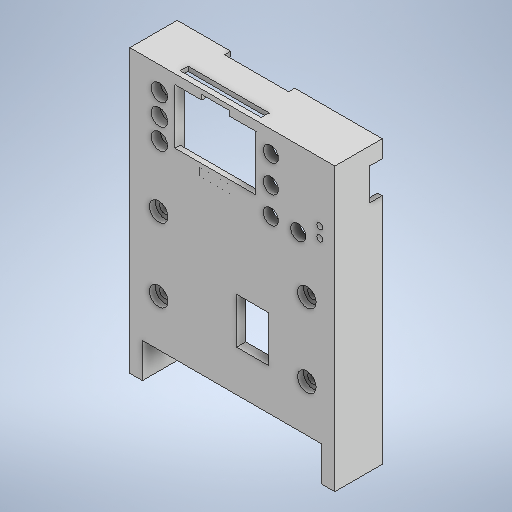
# Autodesk Inventor part: TES_Controller_V1_Case_Top
Saved by Autodesk Inventor 2025 (Build 290162000, 162)
## iProperties
Created: 2025-08-31
Part Number: TES_Controller_V1_Case_Top
Material: 常规
Document SubType Name: Modeling
Designer: 95052
Density: 1 g/cm^3
Appearance: 默认
Author: 95052
Autodesk Inventor part; units mm, degrees
ref_plane "YZ Plane" through (0, 0, 0) normal (1, 0, 0) x (0, 1, 0)
ref_plane "XZ Plane" through (0, 0, 0) normal (0, 1, 0) x (-1, 0, 0)
ref_plane "XY Plane" through (0, 0, 0) normal (0, 0, 1) x (1, 0, 0)
sketch "草图22" plane through (0, 0, 0) normal (0, 0, 1) x (1, 0, 0)
  line L0 (32.055, -44.6465) -> (-32.055, -44.6465)
  line L1 (-32.055, -44.6465) -> (-32.055, 44.6465)
  line L2 (-32.055, 44.6465) -> (32.055, 44.6465)
  line L3 (32.055, 44.6465) -> (32.055, -44.6465)
  line L4 (32.055, -44.6465) -> (-32.055, 44.6465) construction
  line L5 (-32.055, -44.6465) -> (32.055, 44.6465) construction
  line L6 (24.394, -19.5595) -> (-24.107, -19.5595) construction
  line L7 (-24.107, -19.5595) -> (-24.107, 4.4405) construction
  line L8 (-24.107, 4.4405) -> (24.394, 4.4405) construction
  line L9 (24.394, 4.4405) -> (24.394, -19.5595) construction
  line L10 (24.394, -19.5595) -> (-24.107, 4.4405) construction
  line L11 (-24.107, -19.5595) -> (24.394, 4.4405) construction
  circle A0 centre (-24.107, 4.4405) radius 1.7
  circle A1 centre (-24.107, -19.5595) radius 1.7
  circle A2 centre (24.394, -19.5595) radius 1.7
  circle A3 centre (24.394, 4.4405) radius 1.7
  point P0 (0, 0)
  point P1 (-14.525, 44.6465)
  point P2 (3.476, 44.6465)
  point P3 (0.1435, -7.5595)
  dimension "d101" = 89.293
  dimension "d102" = 64.11
  dimension "d103" = 7.661
  dimension "d104" = 7.948
  dimension "d105" = 25.087
  dimension "d106" = 40.206
  dimension "d107" = 17.53
  dimension "d108" = 28.579
  dimension "d109" = 3.4
  dimension "d110" = 3.4
  dimension "d111" = 3.4
  dimension "d112" = 3.4
  constraints: 24 end point, 4 centre point, 4 coincident, 4 midpoint, 4 parallel, 2 horizontal, 2 perpendicular, 2 point on line
  measures "d101" distance of L2.end L0.start
  measures "d102" distance of L0.start L0.end
  measures "d103" distance between parallel lines of L3 L9
  measures "d104" distance between parallel lines of L1 L7
  measures "d105" distance between parallel lines of L0 L6
  measures "d106" distance between parallel lines of L2 L8
  measures "d107" distance from line of L1 point (-14.525, 44.646)
  measures "d108" distance from line of L3 point (3.476, 44.646)
  measures "d109" diameter of A0
  measures "d110" diameter of A1
  measures "d111" diameter of A2
  measures "d112" diameter of A3
extrude "拉伸18" add sketch "草图22" along normal blind 1
sketch "草图23" plane through (0, 0, 1) normal (0, 0, 1) x (1, 0, 0)
  circle A0 centre (-24.107, 4.4405) radius 1.7 projected
  circle A1 centre (24.394, 4.4405) radius 1.7 projected
  circle A2 centre (24.394, -19.5595) radius 1.7 projected
  circle A3 centre (-24.107, -19.5595) radius 1.7 projected
  line L0 (32.055, 44.6465) -> (-32.055, 44.6465) projected
  line L1 (-32.055, -44.6465) -> (32.055, -44.6465) projected
  line L2 (-32.055, 44.6465) -> (32.055, 44.6465)
  line L3 (32.055, 44.6465) -> (32.055, -44.6465)
  line L4 (32.055, -44.6465) -> (-32.055, -44.6465)
  line L5 (-32.055, -44.6465) -> (-32.055, 44.6465)
  circle A4 centre (24.394, 4.4405) radius 3.05
  circle A5 centre (24.394, -19.5595) radius 1.7 projected
  circle A6 centre (24.394, -19.5595) radius 3.05
  circle A7 centre (-24.107, -19.5595) radius 3.05
  circle A8 centre (-24.107, 4.4405) radius 3.05
  point P0 (0, 0)
  dimension "d164" = 6.1
  constraints: 8 coincident, 8 end point, 4 centre point, 3 equal radius, 2 parallel, 1 horizontal, 1 perpendicular
  measures "d164" diameter of A4
extrude "拉伸19" add sketch "草图23" along normal blind 2 contours L3 L1 L5 L0
sketch "草图25" plane through (0, 0, 3) normal (0, 0, 1) x (1, 0, 0)
  circle A0 centre (-23.869, 38.3445) radius 2.7
  circle A1 centre (-23.869, 31.3595) radius 2.7
  circle A2 centre (-23.869, 24.5015) radius 2.7
  line L0 (32.055, 44.6465) -> (-32.055, 44.6465) projected
  line L1 (-32.055, 44.6465) -> (-32.055, -44.6465) projected
  circle A3 centre (12.608, 39.1095) radius 2.5
  line L2 (32.055, -44.6465) -> (32.055, 44.6465) projected
  circle A4 centre (12.608, 30.2185) radius 2.5
  circle A5 centre (12.608, 21.3885) radius 2.5
  circle A6 centre (21.582, 21.3885) radius 2.5
  circle A7 centre (28.639, 26.6255) radius 1
  circle A8 centre (28.639, 23.2155) radius 1
  line L3 (7.225, 20.5575) -> (-18.275, 20.5575) construction
  line L4 (-18.275, 20.5575) -> (-18.275, 47.0575) construction
  line L5 (-18.275, 47.0575) -> (7.225, 47.0575) construction
  line L6 (7.225, 47.0575) -> (7.225, 20.5575) construction
  line L7 (-18.775, 25.0575) -> (7.725, 25.0575)
  line L8 (7.725, 25.0575) -> (7.725, 43.0575)
  line L9 (-18.775, 43.0575) -> (-18.775, 25.0575)
  line L10 (-10.025, 43.0575) -> (-10.025, 47.0575)
  line L11 (-10.025, 47.0575) -> (-5.525, 47.0575)
  line L12 (-1.025, 43.0575) -> (-1.025, 47.0575)
  line L13 (-1.025, 47.0575) -> (-5.525, 47.0575)
  line L14 (7.725, 43.0575) -> (-1.025, 43.0575)
  line L15 (-10.025, 43.0575) -> (-18.775, 43.0575)
  point P0 (0, 0)
  point P1 (-5.525, 21.0575)
  point P2 (-5.525, 20.5575)
  dimension "d123" = 5.4
  dimension "d124" = 5.4
  dimension "d125" = 5.4
  dimension "d126" = 6.302
  dimension "d127" = 8.186
  dimension "d128" = 8.186
  dimension "d129" = 8.186
  dimension "d130" = 13.287
  dimension "d131" = 20.145
  dimension "d132" = 5.537
  dimension "d133" = 19.447
  dimension "d134" = 5
  dimension "d135" = 5
  dimension "d136" = 14.428
  dimension "d137" = 19.447
  dimension "d138" = 5
  dimension "d139" = 19.447
  dimension "d140" = 23.258
  dimension "d141" = 5
  dimension "d142" = 23.258
  dimension "d143" = 10.473
  dimension "d144" = 2
  dimension "d145" = 2
  dimension "d146" = 3.416
  dimension "d147" = 3.416
  dimension "d148" = 18.021
  dimension "d149" = 3.41
  dimension "d150" = 26.53
  dimension "d151" = 23.589
  dimension "d152" = 0.5
  dimension "d153" = 26.53
  dimension "d154" = 26.5
  dimension "d155" = 25.5
  dimension "d156" = 4.5
  dimension "d158" = 0.5
  dimension "d159" = 0.5
  constraints: 26 end point, 9 centre point, 5 parallel, 2 collinear, 2 horizontal, 2 perpendicular, 1 midpoint
  measures "d123" diameter of A0
  measures "d124" diameter of A1
  measures "d125" diameter of A2
  measures "d126" distance from line of L0 A0.centre
  measures "d127" distance from line of L1 A0.centre
  measures "d128" distance from line of L1 A1.centre
  measures "d129" distance from line of L1 A2.centre
  measures "d130" distance from line of L0 A1.centre
  measures "d131" distance from line of L0 A2.centre
  measures "d132" distance from line of L0 A3.centre
  measures "d133" distance from line of L2 A3.centre
  measures "d134" diameter of A3
  measures "d135" diameter of A4
  measures "d136" distance from line of L0 A4.centre
  measures "d137" distance from line of L2 A4.centre
  measures "d138" diameter of A5
  measures "d139" distance from line of L2 A5.centre
  measures "d140" distance from line of L0 A5.centre
  measures "d141" diameter of A6
  measures "d142" distance from line of L0 A6.centre
  measures "d143" distance from line of L2 A6.centre
  measures "d144" diameter of A7
  measures "d145" diameter of A8
  measures "d146" distance from line of L2 A7.centre
  measures "d147" distance from line of L2 A8.centre
  measures "d148" distance from line of L0 A7.centre
  measures "d149" distance of A7.centre A8.centre
  measures "d150" distance from line of L1 point (-5.525, 21.058)
  measures "d151" distance from line of L0 point (-5.525, 21.058)
  measures "d152" distance from line of point (-5.525, 21.058) L3
  measures "d153" distance from line of L1 point (-5.525, 20.558)
  measures "d154" distance of L3.end L4.end
  measures "d155" distance of L3.start L3.end
  measures "d156" distance between parallel lines of L3 L7
  measures "d158" distance between parallel lines of L4 L9
  measures "d159" distance between parallel lines of L6 L8
extrude "拉伸21" cut sketch "草图25" against normal up to next
sketch "草图26" plane through (0, 0, 3) normal (0, 0, 1) x (1, 0, 0)
  circle A0 centre (-24.107, 4.4405) radius 1.7 projected
  circle A1 centre (-24.107, -19.5595) radius 1.7 projected
  circle A2 centre (24.394, 4.4405) radius 1.7 projected
  circle A3 centre (24.394, -19.5595) radius 1.7 projected
  line L0 (1.394, -6.2595) -> (11.894, -6.2595)
  line L1 (11.894, -6.2595) -> (11.894, -21.2595)
  line L2 (11.894, -21.2595) -> (1.394, -21.2595)
  line L3 (1.394, -21.2595) -> (1.394, -6.2595)
  line L4 (-24.107, -19.5595) -> (24.394, -19.5595) construction
  line L5 (32.055, -44.6465) -> (32.055, 44.6465) construction
  line L6 (24.394, -21.2595) -> (-24.107, -21.2595) construction
  point P0 (0, 0)
  dimension "d165" = 12.5
  dimension "d166" = 23
  dimension "d167" = 15
  constraints: 12 end point, 2 horizontal, 2 parallel, 2 perpendicular, 2 vertical alignment, 1 collinear, 2 other
  measures "d165" distance from line of L1 L4.end
  measures "d166" distance from line of L4.end L3
  measures "d167" distance between parallel lines of L2 L0
extrude "拉伸22" cut sketch "草图26" against normal through all contours L0 L1 L2 L3
sketch "草图27" plane through (0, 0, 0) normal (0, 0, -1) x (-1, 0, 0)
  line L0 (10.855, 21.0575) -> (0.195, 21.0575)
  line L1 (0.195, 21.0575) -> (0.195, 23.5575)
  line L2 (0.195, 23.5575) -> (10.855, 23.5575)
  line L3 (10.855, 23.5575) -> (10.855, 21.0575)
  line L4 (10.025, 44.6465) -> (32.055, 44.6465) projected
  line L5 (32.055, 44.6465) -> (32.055, -44.6465) projected
  point P0 (0, 0)
  dimension "d170" = 23.589
  dimension "d171" = 21.089
  dimension "d172" = 21.2
  dimension "d173" = 31.86
  constraints: 8 end point, 2 parallel, 1 horizontal, 1 perpendicular
  measures "d170" distance between parallel lines of L4 L0
  measures "d171" distance between parallel lines of L4 L2
  measures "d172" distance between parallel lines of L5 L3
  measures "d173" distance between parallel lines of L5 L1
extrude "拉伸23" cut sketch "草图27" against normal blind 2.8
sketch "草图28" plane through (0, 0, 3) normal (0, 0, 1) x (1, 0, 0)
  line L0 (-32.055, -44.6465) -> (32.055, -44.6465) projected
  line L1 (-29.408, -44.6465) -> (29.212, -44.6465)
  line L2 (29.212, -44.6465) -> (29.212, -34.7635)
  line L3 (29.212, -34.7635) -> (-29.408, -34.7635)
  line L4 (-29.408, -34.7635) -> (-29.408, -44.6465)
  line L5 (32.055, -44.6465) -> (32.055, 44.6465) projected
  line L6 (-32.055, 44.6465) -> (-32.055, -44.6465) projected
  point P0 (0, 0)
  point P1 (29.212, -44.6465)
  dimension "d176" = 2.843
  dimension "d177" = 2.647
  dimension "d178" = 9.883
  constraints: 8 end point, 2 parallel, 1 horizontal, 1 perpendicular, 1 point on line
  measures "d176" distance between parallel lines of L2 L5
  measures "d177" distance between parallel lines of L6 L4
  measures "d178" distance between parallel lines of L0 L3
extrude "拉伸24" cut sketch "草图28" against normal through all
sketch "草图29" plane through (0, 0, 0) normal (0, 0, -1) x (-1, 0, 0)
  line L0 (29.408, -34.7635) -> (-29.212, -34.7635) projected
  line L1 (29.408, -34.7635) -> (-29.212, -34.7635)
  line L2 (-29.212, -34.7635) -> (-29.212, -32.7635)
  line L3 (-29.212, -32.7635) -> (29.408, -32.7635)
  line L4 (29.408, -32.7635) -> (29.408, -34.7635)
  point P0 (0, 0)
  point P1 (-29.212, -34.7635)
  dimension "d181" = 2
  constraints: 8 end point, 2 parallel, 1 horizontal, 1 perpendicular
  measures "d181" distance of L1.end L2.end
extrude "拉伸25" add sketch "草图29" along normal blind 3
sketch "草图30" plane through (0, 0, 0) normal (0, 0, -1) x (-1, 0, 0)
  line L0 (29.408, -32.7635) -> (29.408, -34.7635) projected
  line L1 (32.055, 44.6465) -> (32.055, -44.6465) projected
  line L2 (29.408, -32.7635) -> (32.055, -32.7635)
  line L3 (32.055, -32.7635) -> (32.055, -44.6465)
  line L4 (32.055, -44.6465) -> (29.408, -44.6465)
  line L5 (29.408, -44.6465) -> (29.408, -32.7635)
  line L6 (-29.212, -34.7635) -> (-29.212, -32.7635) projected
  line L7 (-32.055, -44.6465) -> (-32.055, 44.6465) projected
  line L8 (-29.212, -32.7635) -> (-32.055, -32.7635)
  line L9 (-32.055, -32.7635) -> (-32.055, -44.6465)
  line L10 (-32.055, -44.6465) -> (-29.212, -44.6465)
  line L11 (-29.212, -44.6465) -> (-29.212, -32.7635)
  point P0 (0, 0)
  constraints: 16 end point, 4 parallel, 2 horizontal, 2 perpendicular
extrude "拉伸26" add sketch "草图30" along normal blind 11.5
sketch "草图31" plane through (0, 0, 0) normal (0, 0, -1) x (-1, 0, 0)
  line L0 (-32.055, -32.7635) -> (-32.055, 44.6465) projected
  line L1 (32.055, 44.6465) -> (32.055, -32.7635) projected
  line L2 (-33.555, 44.6465) -> (-33.555, -44.6465)
  line L3 (-32.055, -44.6465) -> (-32.055, 44.6465)
  line L4 (33.555, 44.6465) -> (33.555, -44.6465)
  line L5 (32.055, -44.6465) -> (32.055, 44.6465)
  line L6 (-32.055, 44.6465) -> (32.055, 44.6465)
  line L7 (33.555, 44.6465) -> (33.555, 46.1465)
  line L8 (33.555, 46.1465) -> (-33.555, 46.1465)
  line L9 (-33.555, 46.1465) -> (-33.555, 44.6465)
  line L10 (29.408, -44.6465) -> (32.055, -44.6465)
  line L11 (33.555, -44.6465) -> (33.555, -46.1465)
  line L12 (33.555, -46.1465) -> (29.408, -46.1465)
  line L13 (29.408, -46.1465) -> (29.408, -44.6465)
  line L14 (-32.055, -44.6465) -> (-29.212, -44.6465)
  line L15 (-29.212, -44.6465) -> (-29.212, -46.1465)
  line L16 (-29.212, -46.1465) -> (-33.555, -46.1465)
  line L17 (-33.555, -46.1465) -> (-33.555, -44.6465)
  point P0 (0, 0)
  point P1 (-32.055, 44.6465)
  point P2 (32.055, -32.7635)
  dimension "d188" = 1.5
  dimension "d202" = 1.5
  constraints: 32 end point, 8 parallel, 3 horizontal, 3 perpendicular, 3 point on line
  measures "d188" distance of L7.end L7.start
  measures "d202" distance of L14.end L15.end
extrude "拉伸27" add sketch "草图31" along normal blind 11.5 and the other way blind 3
sketch "草图32" plane through (-33.555, 46.1465, -11.5) normal (0, 1, 0) x (1, 0, 0)
  line L0 (14.78, -11.5) -> (41.28, -11.5) projected
  line L1 (41.28, -11.5) -> (14.78, -11.5)
  line L2 (14.78, -11.5) -> (14.78, -10.2)
  line L3 (14.78, -10.2) -> (41.28, -10.2)
  line L4 (41.28, -10.2) -> (41.28, -11.5)
  point P0 (33.555, -11.5)
  dimension "d193" = 1.3
  constraints: 8 end point, 2 parallel, 1 horizontal, 1 perpendicular
  measures "d193" distance of L1.end L2.end
extrude "拉伸28" cut sketch "草图32" against normal blind 11
sketch "草图33" plane through (-33.555, 46.1465, -11.5) normal (0, 1, 0) x (1, 0, 0)
  line L0 (65.61, 0) -> (1.5, 0) projected
  line L1 (17.53, 0) -> (38.5, 0)
  line L2 (38.5, 0) -> (38.5, -1)
  line L3 (38.5, -1) -> (17.53, -1)
  line L4 (17.53, -1) -> (17.53, 0)
  point P0 (33.555, -11.5)
  dimension "d196" = 16.03
  dimension "d197" = 37
  dimension "d198" = 1
  constraints: 8 end point, 2 parallel, 1 horizontal, 1 perpendicular, 1 point on line
  measures "d196" distance from line of L4 L0.end
  measures "d197" distance from line of L0.end L2
  measures "d198" distance between parallel lines of L0 L3
extrude "拉伸29" cut sketch "草图33" against normal blind 11
sketch "草图34" plane through (0, 0, 0) normal (0, 0, -1) x (-1, 0, 0)
  line L0 (18.775, 44.6465) -> (32.055, 44.6465) projected
  line L1 (18.775, 21.0575) -> (18.775, 44.6465)
  line L2 (-7.725, 44.6465) -> (-7.725, 21.0575)
  line L3 (10.855, 21.0575) -> (0.195, 21.0575) projected
  line L4 (18.775, 20.5575) -> (-7.725, 20.5575)
  line L5 (-7.725, 46.1465) -> (18.775, 46.1465)
  line L6 (-7.725, 44.6465) -> (-7.725, 46.1465)
  line L7 (-7.725, 46.1465) -> (-7.725, 44.6465) projected
  line L8 (-7.725, 21.0575) -> (-7.725, 20.5575)
  line L9 (18.775, 21.0575) -> (18.775, 20.5575)
  line L10 (18.775, 44.6465) -> (18.775, 46.1465)
  line L11 (-4.945, 46.1465) -> (16.025, 46.1465) projected
  point P0 (0, 0)
  constraints: 16 end point, 3 point on line, 2 parallel, 1 collinear, 1 perpendicular
extrude "拉伸30" cut sketch "草图34" against normal blind 1.3
sketch "草图35" plane through (33.555, -46.1465, -11.5) normal (1, 0, 0) x (0, 0, -1)
  line L0 (0, 90.793) -> (0, 13.383) projected
  line L1 (0, 86.614) -> (-3, 86.614)
  line L2 (-3, 86.614) -> (-3, 76.174)
  line L3 (-3, 76.174) -> (0, 76.174)
  line L4 (0, 76.174) -> (0, 86.614)
  line L5 (-11.5, 90.793) -> (0, 90.793) projected
  point P0 (-11.5, 46.1465)
  point P1 (-1.5, 86.614)
  point P2 (0, 76.174)
  point P3 (-0.0335, 85.614)
  dimension "d206" = 4.179
  dimension "d207" = 14.619
  dimension "d208" = 3
  constraints: 8 end point, 2 parallel, 1 horizontal, 1 midpoint, 1 perpendicular, 1 point on line
  measures "d206" distance from line of L5 point (-1.5, 86.614)
  measures "d207" distance between parallel lines of L5 L3
  measures "d208" distance between parallel lines of L0 L2
extrude "拉伸31" cut sketch "草图35" against normal up to surface (1.5 mm away)
sketch "草图37" plane through (0, 0, 0) normal (0, 0, -1) x (-1, 0, 0)
  circle A0 centre (24.107, 4.4405) radius 1.7 projected
  circle A1 centre (24.107, 4.4405) radius 3
  circle A2 centre (24.107, -19.5595) radius 1.7 projected
  circle A3 centre (24.107, -19.5595) radius 3
  circle A4 centre (-24.394, 4.4405) radius 1.7 projected
  circle A5 centre (-24.394, 4.4405) radius 3
  circle A6 centre (-24.394, -19.5595) radius 1.7 projected
  circle A7 centre (-24.394, -19.5595) radius 3
  point P0 (0, 0)
  dimension "d213" = 6
  dimension "d214" = 6
  dimension "d215" = 6
  dimension "d216" = 6
  constraints: 4 centre point, 4 coincident
  measures "d213" diameter of A1
  measures "d214" diameter of A3
  measures "d215" diameter of A5
  measures "d216" diameter of A7
extrude "拉伸33" add sketch "草图37" along normal blind 0.5
sketch "草图38" plane through (0, 0, -11.5) normal (0, 0, -1) x (-1, 0, 0)
  line L0 (-33.555, 30.0275) -> (-33.555, -46.1465) projected
  line L1 (-33.555, -46.1465) -> (-29.212, -46.1465) projected
  line L2 (-29.212, -46.1465) -> (-29.212, -32.7635) projected
  line L3 (-29.212, -32.7635) -> (-32.055, -32.7635) projected
  line L4 (-32.055, -32.7635) -> (-32.055, 30.0275) projected
  line L5 (-32.055, 30.0275) -> (-33.555, 30.0275) projected
  line L6 (-33.555, 40.4675) -> (-32.055, 40.4675) projected
  line L7 (-32.055, 40.4675) -> (-32.055, 44.6465) projected
  line L8 (-33.555, 46.1465) -> (-33.555, 40.4675) projected
  line L9 (-33.555, 40.4675) -> (-32.055, 40.4675) projected
  line L10 (-32.055, 40.4675) -> (-32.055, 44.6465) projected
  line L11 (-32.055, 44.6465) -> (-4.945, 44.6465) projected
  line L12 (-4.945, 44.6465) -> (-4.945, 46.1465) projected
  line L13 (-4.945, 46.1465) -> (-33.555, 46.1465) projected
  line L14 (-33.555, 46.1465) -> (-33.555, 40.4675) projected
  line L15 (16.025, 46.1465) -> (16.025, 44.6465) projected
  line L16 (16.025, 44.6465) -> (32.055, 44.6465) projected
  line L17 (32.055, 44.6465) -> (32.055, -32.7635) projected
  line L18 (32.055, -32.7635) -> (29.408, -32.7635) projected
  line L19 (29.408, -32.7635) -> (29.408, -46.1465) projected
  line L20 (29.408, -46.1465) -> (33.555, -46.1465) projected
  line L21 (33.555, -46.1465) -> (33.555, 46.1465) projected
  line L22 (33.555, 46.1465) -> (16.025, 46.1465) projected
  point P0 (0, 0)
extrude "拉伸34" add sketch "草图38" along normal blind 1
